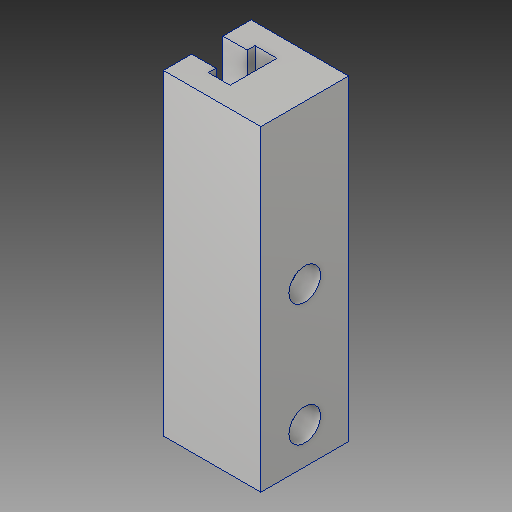
# Autodesk Inventor part: HeadbarHolderBracketAdjustable20mm
Saved by Autodesk Inventor 2019 (Build 230136000, 136)
## iProperties
Created: 2015-11-11
Part Number: HeadbarHolderBracketAdjustable20mm
Material: Aluminum 6061
Document SubType Name: Modeling
Designer: runeala
Mass: 58.2626 g
Surface Area: 83.753 cm^2
Volume: 21.5787 cm^3
Density: 2.7 g/cm^3
Appearance: Aluminum - Flat
Author: runeala
Autodesk Inventor part; units mm, degrees
ref_plane "YZ Plane" through (0, 0, 0) normal (1, 0, 0) x (0, 1, 0)
ref_plane "XZ Plane" through (0, 0, 0) normal (0, 1, 0) x (-1, 0, 0)
ref_plane "XY Plane" through (0, 0, 0) normal (0, 0, 1) x (1, 0, 0)
sketch "Sketch1" plane through (0, 0, 0) normal (0, 1, 0) x (-1, 0, 0)
  line L0 (0, 0) -> (20, 0)
  line L1 (20, 0) -> (20, 18)
  line L2 (20, 18) -> (0, 18)
  line L3 (0, 18) -> (0, 0)
  dimension "d0" = 18
  dimension "d1" = 20
  constraints: 8 end point, 2 parallel, 1 horizontal, 1 perpendicular
  measures "d0" distance of L0.end L1.end
  measures "d1" distance of L1.end L2.end
extrude "Extrusion1" add sketch "Sketch1" along normal mid plane 65
sketch "Sketch2" plane through (-20, -32.5, 18) normal (-1, 0, 0) x (0, 0, 1)
  circle A0 centre (-9, 7.5) radius 3.25
  circle A1 centre (-9, 32.5) radius 3.25
  circle A2 centre (-9, 7.5) radius 5.5
  circle A3 centre (-9, 32.5) radius 5.5
  line L0 (0, 0) -> (-18, 0) projected
  line L1 (-18, 32.5) -> (8.866, 32.5) construction
  line L2 (-9, 65.0931) -> (-9, 0) construction
  dimension "d4" = 6.5
  dimension "d5" = 6.5
  dimension "d8" = 11
  dimension "d9" = 11
  dimension "d34" = 25
  constraints: 4 centre point, 4 end point, 2 coincident, 2 point on line, 1 horizontal, 1 midpoint
  measures "d4" diameter of A0
  measures "d5" diameter of A1
  measures "d8" diameter of A2
  measures "d9" diameter of A3
  measures "d34" distance of A1.centre A0.centre
extrude "Extrusion2" cut sketch "Sketch2" against normal through all contours A0 | A1
extrude "Extrusion3" cut sketch "Sketch2" against normal blind 15.5
sketch "Sketch4" plane through (0, 32.5, 0) normal (0, 1, 0) x (1, 0, 0)
  line L0 (-20, 0) -> (-20, -18) projected
  line L1 (-20, -9) -> (2.4786, -9) construction
  line L2 (-20, -12.2) -> (-15, -12.2)
  line L3 (-15, -12.2) -> (-15, -13.8)
  line L4 (-15, -13.8) -> (-10.5, -13.8)
  line L5 (-10.5, -13.8) -> (-10.5, -4.2)
  line L6 (-10.5, -4.2) -> (-15, -4.2)
  line L7 (-15, -4.2) -> (-15, -5.8)
  line L8 (-15, -5.8) -> (-20, -5.8)
  line L9 (-20, -12.2) -> (-20, -5.8)
  point P0 (0, 0)
  dimension "d28" = 6.4
  dimension "d29" = 4.5
  dimension "d30" = 9.6
  dimension "d31" = 5
  constraints: 18 end point, 4 perpendicular, 4 point on line, 2 horizontal, 1 collinear, 1 midpoint, 2 other
  measures "d28" distance between parallel lines of L8 L2
  measures "d29" distance of L5.end L6.end
  measures "d30" distance of L4.end L5.end
  measures "d31" distance of L2.start L2.end
extrude "Extrusion4" cut sketch "Sketch4" against normal through all
body "Solid1"
